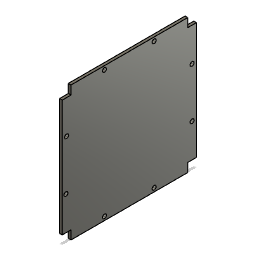
Боковые стенки Cubesatb 3.0 v8 (Autodesk Fusion 360 design; units mm, degrees)
Autodesk Fusion 360 part; units mm, degrees
note: some values were not read from the file. Set by a fixed rule: which sketch regions a step uses.
sketch "Sketch1" plane through (0, 0, 0) normal (1, 0, 0) x (0, 0, -1)
  line L0 (0, 0) -> (-100, 0)
  line L1 (-100, 0) -> (-100, 100)
  line L2 (-100, 100) -> (0, 100)
  line L3 (0, 100) -> (0, 0)
  dimension "d1" = 100
  dimension "d2" = 100
  constraint horizontal L0
  constraint vertical L1
  constraint horizontal L2
  constraint vertical L3
  constraint coincident L0.start L3.end
  measures "d1" distance of L0.start L0.end
  measures "d2" distance of L0.start L2.end
extrude "Extrude1" add sketch "Sketch1" against normal blind 2
extrude "Extrude2" add 1 faces at (0, 33.3333, 33.3333) along direction (1, 0, 0) blind 2
extrude "Extrude3" add 1 faces at (2, 33.3333, 33.3333) along direction (1, 0, 0) blind 1
sketch "Sketch2" plane through (3, 0, 0) normal (1, 0, 0) x (0, 0, -1)
  line L0 (-100, 100) -> (0, 100)
  line L1 (0, 100) -> (0, 0)
  line L2 (0, 0) -> (-100, 0)
  line L3 (-100, 0) -> (-100, 100)
  line L4 (-100, 100) -> (-68.5, 100)
  line L5 (-68.5, 100) -> (-68.5, 94.5)
  line L6 (-68.5, 94.5) -> (-100, 94.5)
  line L7 (-100, 94.5) -> (-100, 100)
  line L8 (-100, 100) -> (-93.5, 100)
  line L9 (-93.5, 100) -> (-93.5, 68.5)
  line L10 (0, 100) -> (-6.5, 100)
  line L11 (-6.5, 100) -> (-6.5, 68.5)
  line L12 (-6.5, 68.5) -> (0, 68.5)
  line L13 (0, 68.5) -> (0, 100)
  line L14 (0, 100) -> (-31.5, 100)
  line L15 (-31.5, 100) -> (-31.5, 94.5)
  line L16 (-31.5, 94.5) -> (0, 94.5)
  line L17 (0, 94.5) -> (0, 100)
  line L18 (0, 0) -> (-6.5, 0)
  line L19 (-6.5, 0) -> (-6.5, 31.5)
  line L20 (-6.5, 31.5) -> (0, 31.5)
  line L21 (0, 31.5) -> (0, 0)
  line L22 (0, 0) -> (-31.5, 0)
  line L23 (-31.5, 0) -> (-31.5, 5.5)
  line L24 (-31.5, 5.5) -> (0, 5.5)
  line L25 (0, 5.5) -> (0, 0)
  line L26 (-100, 0) -> (-68.5, 0)
  line L27 (-68.5, 0) -> (-68.5, 5.5)
  line L28 (-68.5, 5.5) -> (-100, 5.5)
  line L29 (-100, 5.5) -> (-100, 0)
  line L30 (-100, 0) -> (-94.5, 0)
  line L31 (-94.5, 0) -> (-94.5, 31.5)
  line L32 (-94.5, 31.5) -> (-100, 31.5)
  line L33 (-100, 31.5) -> (-100, 0)
  circle A0 centre (-68.5, 97.25) radius 1.5
  circle A1 centre (-97.25, 31.5) radius 1.5
  circle A2 centre (-68.5, 2.75) radius 1.5
  circle A3 centre (-31.5, 2.75) radius 1.5
  circle A4 centre (-3.25, 31.5) radius 1.5
  circle A5 centre (-3.25, 68.5) radius 1.5
  circle A6 centre (-31.5, 97.25) radius 1.5
  line L34 (-93.5, 68.5) -> (-100, 68.5)
  line L35 (-100, 68.5) -> (-100, 100)
  line L36 (-100, 100) -> (-93.5, 100)
  line L37 (-93.5, 100) -> (-93.5, 68.5)
  circle A7 centre (-96.75, 68.5) radius 1.5
  line L38 (-100, 100) -> (-93.5, 100)
  line L39 (-93.5, 100) -> (-93.5, 93.5)
  line L40 (-93.5, 93.5) -> (-100, 93.5)
  line L41 (-100, 93.5) -> (-100, 100)
  line L42 (-100, 0) -> (-93.5, 0)
  line L43 (-93.5, 0) -> (-93.5, 6.5)
  line L44 (-93.5, 6.5) -> (-100, 6.5)
  line L45 (-100, 6.5) -> (-100, 0)
  line L46 (0, 0) -> (-6.5, 0)
  line L47 (-6.5, 0) -> (-6.5, 6.5)
  line L48 (-6.5, 6.5) -> (0, 6.5)
  line L49 (0, 6.5) -> (0, 0)
  line L50 (0, 100) -> (-6.5, 100)
  line L51 (-6.5, 100) -> (-6.5, 93.5)
  line L52 (-6.5, 93.5) -> (0, 93.5)
  line L53 (0, 93.5) -> (0, 100)
  dimension "d53" = 31.5
  dimension "d54" = 5.5
  dimension "d55" = 6.5
  dimension "d57" = 6.5
  dimension "d58" = 31.5
  dimension "d59" = 31.5
  dimension "d60" = 5.5
  dimension "d61" = 6.5
  dimension "d62" = 31.5
  dimension "d63" = 5.5
  dimension "d64" = 31.5
  dimension "d65" = 5.5
  dimension "d66" = 31.5
  dimension "d67" = 100
  dimension "d68" = 100
  dimension "d69" = 5.5
  dimension "d70" = 31.5
  dimension "d71" = 3
  dimension "d73" = 3
  dimension "d74" = 3
  dimension "d75" = 3
  dimension "d76" = 3
  dimension "d77" = 3
  dimension "d78" = 3
  dimension "d81" = 31.5
  dimension "d83" = 3
  dimension "d88" = 6.5
  dimension "d89" = 6.5
  dimension "d90" = 6.5
  dimension "d91" = 6.5
  dimension "d92" = 6.5
  dimension "d93" = 6.5
  dimension "d94" = 6.5
  dimension "d95" = 6.5
  constraint horizontal L0
  constraint vertical L1
  constraint horizontal L2
  constraint vertical L3
  constraint coincident L1.end L2.start
  constraint horizontal L4
  constraint vertical L5
  constraint horizontal L6
  constraint vertical L7
  constraint horizontal L8
  constraint vertical L9
  constraint horizontal L10
  constraint vertical L11
  constraint horizontal L12
  constraint vertical L13
  constraint horizontal L14
  constraint vertical L15
  constraint horizontal L16
  constraint vertical L17
  constraint horizontal L18
  constraint vertical L19
  constraint horizontal L20
  constraint vertical L21
  constraint horizontal L22
  constraint vertical L23
  constraint horizontal L24
  constraint vertical L25
  constraint horizontal L26
  constraint vertical L27
  constraint horizontal L28
  constraint vertical L29
  constraint horizontal L30
  constraint vertical L31
  constraint horizontal L32
  constraint vertical L33
  constraint midpoint L5 A0.centre
  constraint midpoint L32 A1.centre
  constraint midpoint L27 A2.centre
  constraint midpoint L23 A3.centre
  constraint midpoint L20 A4.centre
  constraint midpoint L12 A5.centre
  constraint midpoint L15 A6.centre
  constraint horizontal L34
  constraint vertical L35
  constraint horizontal L36
  constraint vertical L37
  constraint midpoint L34 A7.centre
  constraint horizontal L38
  constraint vertical L39
  constraint horizontal L40
  constraint vertical L41
  constraint horizontal L42
  constraint vertical L43
  constraint horizontal L44
  constraint vertical L45
  constraint horizontal L46
  constraint vertical L47
  constraint horizontal L48
  constraint vertical L49
  constraint horizontal L50
  constraint vertical L51
  constraint horizontal L52
  constraint vertical L53
  measures "d53" distance of L0.start L4.end
  measures "d54" distance of L0.start L6.end
  measures "d55" distance of L0.start L8.end
  measures "d57" distance of L0.end L10.end
  measures "d58" distance of L0.end L12.end
  measures "d59" distance of L0.end L14.end
  measures "d60" distance of L0.end L16.end
  measures "d61" distance of L1.end L18.end
  measures "d62" distance of L1.end L20.end
  measures "d63" distance of L1.end L24.end
  measures "d64" distance of L2.end L26.end
  measures "d65" distance of L2.end L30.end
  measures "d66" distance of L2.end L32.end
  measures "d67" distance of L3 L13
  measures "d68" distance of L0 L2
  measures "d69" distance of L26 L28
  measures "d70" distance of L23 L25
  measures "d71" diameter of A0
  measures "d73" diameter of A1
  measures "d74" diameter of A2
  measures "d75" diameter of A3
  measures "d76" diameter of A4
  measures "d77" diameter of A5
  measures "d78" diameter of A6
  measures "d81" distance of L8 L34
  measures "d83" diameter of A7
  measures "d88" distance of L0.start L8.end
  measures "d89" distance of L0.start L40.end
  measures "d90" distance of L2.end L42.end
  measures "d91" distance of L2.end L44.end
  measures "d92" distance of L1.end L18.end
  measures "d93" distance of L1.end L48.end
  measures "d94" distance of L0.end L10.end
  measures "d95" distance of L0.end L52.end
extrude "Extrude9" cut sketch "Sketch2" against normal blind 20 contours L5 A0 | L5 A0 | L15 A6 | L15 A6 | L34 A7 | L34 A7 | L32 A1 | L32 A1 | L12 A5 | L12 A5 | L20 A4 | L20 A4 | L27 A2 | L27 A2 | L23 A3 | L23 A3
extrude "Extrude10" cut sketch "Sketch2" against normal blind 3 contours L0 L3 L4 L6 L7 L8 L9 L35 L36 L37 L38 L39 L41 | L0 L4 L5 L6 L9 A0 L37 L39 | L3 L6 L9 L35 L37 L39 L40 L41 | L0 L1 L2 L3 L5 L6 L9 L11 L12 L15 L16 L19 L20 L23 L24 L27 L28 L31 L32 A0 A1 A2 A3 A4 A5 A6 L34 L37 A7 L39 L43 L44 L47 L51 | L3 L9 L34 L35 L37 A7 L40 | L0 L11 L14 L15 L16 A6 L51 | L0 L1 L10 L11 L13 L14 L16 L17 L50 L51 L53 | L3 L31 L32 L33 A1 L44 | L1 L11 L13 L16 L51 L52 L53 | L3 L28 L31 L33 L44 L45 | L1 L11 L12 L13 A5 L52 | L2 L3 L26 L28 L29 L30 L31 L33 L42 L45 | L28 L31 L43 L44 | L2 L26 L28 L31 L42 L43 | L2 L26 L27 L28 A2 L43 | L1 L19 L20 L21 A4 L48 | L1 L19 L21 L24 L47 L48 L49 | L1 L2 L18 L19 L21 L22 L24 L25 L46 L47 L49 | L2 L19 L22 L23 L24 A3 L47
extrude "Extrude11" cut sketch "Sketch2" against normal blind 70 contours L0 L3 L4 L6 L7 L8 L9 L35 L36 L37 L38 L39 L41 | L3 L6 L9 L35 L37 L39 L40 L41 | L0 L1 L10 L11 L13 L14 L16 L17 L50 L51 L53 | L1 L11 L13 L16 L51 L52 L53 | L3 L28 L31 L33 L44 L45 | L2 L3 L26 L28 L29 L30 L31 L33 L42 L45 | L28 L31 L43 L44 | L2 L26 L28 L31 L42 L43 | L1 L19 L21 L24 L47 L48 L49 | L1 L2 L18 L19 L21 L22 L24 L25 L46 L47 L49
